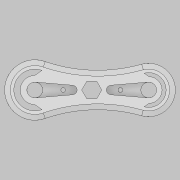
# Autodesk Inventor part: Femur_V2
Saved by Autodesk Inventor 2022.2 (Build 262287010, 287A)
## iProperties
Created: 2022-06-03
Part Number: Femur_V2
Material: Genérico
Document SubType Name: Modeling
Designer: Usuario
Density: 1 g/cm^3
Appearance: Valor por defecto
Author: Usuario
Autodesk Inventor part; units mm, degrees
ref_plane "YZ Plane" through (0, 0, 0) normal (1, 0, 0) x (0, 1, 0)
ref_plane "XZ Plane" through (0, 0, 0) normal (0, 1, 0) x (-1, 0, 0)
ref_plane "XY Plane" through (0, 0, 0) normal (0, 0, 1) x (1, 0, 0)
sketch "Boceto1" plane through (0, 0, 0) normal (0, 1, 0) x (-1, 0, 0)
  arc A0 (20.01, -12.2) -> (20.01, 12.2) centre (24.5, 0) ccw
  arc A1 (-21.2615, 11.0346) -> (-21.2615, -11.0346) centre (-24.5, 0) ccw
  line L0 (-2.1651, 3.75) -> (2.1651, 3.75)
  line L1 (2.1651, 3.75) -> (4.3301, 0)
  line L2 (4.3301, 0) -> (2.1651, -3.75)
  line L3 (2.1651, -3.75) -> (-2.1651, -3.75)
  line L4 (-2.1651, -3.75) -> (-4.3301, 0)
  line L5 (-4.3301, 0) -> (-2.1651, 3.75)
  line L6 (0, 0) -> (0, 8.5) construction
  line L7 (0, 0) -> (0, -8.5) construction
  line L8 (0, 0) -> (2.6275, 0) construction
  arc A2 (20.01, -12.2) -> (-21.4933, -11.1) centre (-2.4996, -77.9761) ccw
  arc A3 (-21.4933, 11.1) -> (20.01, 12.2) centre (-2.4996, 77.9761) ccw
  arc A4 (20.01, 12.2) -> (20.01, -12.2) centre (24.5, 0) ccw construction
  arc A5 (-21.2615, -11.0346) -> (-21.2615, 11.0346) centre (-24.5, 0) ccw construction
  point P0 (-21.4933, 11.1)
  dimension "d2" = 7.5
  dimension "d3" = 49
  dimension "d4" = 8.5
  dimension "d5" = 8.5
  dimension "d6" = 26
  dimension "d7" = 23
  dimension "d12" = 12.2
  dimension "d13" = 11.1
  constraints: 18 end point, 16 point on circle, 6 centre point, 4 symmetric about line, 2 horizontal, 2 vertical, 1 coincident, 14 other
  measures "d2" distance between parallel lines of L0 L3
  measures "d3" distance of A1.centre A0.centre
  measures "d4" distance of L6.start L6.end
  measures "d5" distance of L6.start L7.end
  measures "d6" diameter of A0
  measures "d7" diameter of A1
  measures "d12" vertical distance of A0.centre A0.start
  measures "d13" vertical distance of A1.centre A2.end
extrude "Extrusión1" add sketch "Boceto1" along normal blind 9
sketch "Boceto2" plane through (0, 9, 0) normal (0, 1, 0) x (1, 0, 0)
  arc A0 (-20.01, 12.2) -> (-20.01, -12.2) centre (-24.5, 0) ccw projected
  arc A1 (21.4933, -11.1) -> (21.4933, 11.1) centre (24.5, 0) ccw projected
  arc A2 (-24.5, 6.25) -> (-24.5, -6.25) centre (-24.5, 0) ccw
  arc A3 (24.5, -5.75) -> (24.5, 5.75) centre (24.5, 0) ccw
  arc A4 (-21.3915, 8.4462) -> (-21.3915, -8.4462) centre (-24.5, 0) ccw
  arc A5 (22.5391, -7.2391) -> (22.5391, 7.2391) centre (24.5, 0) ccw
  line L0 (-21.3915, 8.4462) -> (-24.5, 6.25)
  line L1 (-21.3915, -8.4462) -> (-24.5, -6.25)
  arc A6 (-24.5, -6.25) -> (-24.5, 6.25) centre (-24.5, 0) ccw construction
  line L2 (22.5391, 7.2391) -> (24.5, 5.75)
  line L3 (22.5391, -7.2391) -> (24.5, -5.75)
  arc A7 (24.5, 5.75) -> (24.5, -5.75) centre (24.5, 0) ccw construction
  point P0 (0, 0)
  dimension "d16" = 12.5
  dimension "d17" = 11.5
  dimension "d18" = 4
  dimension "d19" = 4
  constraints: 12 point on circle, 8 end point, 6 centre point, 2 coincident
  measures "d16" diameter of A2
  measures "d17" diameter of A3
  measures "d18" radial gap between concentric circles of A0 A4
  measures "d19" radial gap between concentric circles of A1 A5
extrude "Extrusión2" cut sketch "Boceto2" against normal up to surface (9 mm away)
sketch "Boceto3" plane through (0, 9, 0) normal (0, 1, 0) x (1, 0, 0)
  arc A0 (-24.5, 6.25) -> (-24.5, -6.25) centre (-24.5, 0) ccw projected
  arc A1 (24.5, -5.75) -> (24.5, 5.75) centre (24.5, 0) ccw projected
  arc A2 (-24.2158, 3.3881) -> (-24.2158, -3.3881) centre (-24.5, 0) ccw
  arc A3 (-8.1786, -2.0428) -> (-8.1786, 2.0428) centre (-8.35, 0) ccw
  line L0 (-27.9, 3.184) -> (-27.9, -2.3152) construction
  line L1 (-6.3, 2.5123) -> (-6.3, -1.5596) construction
  line L2 (0, 0) -> (0, -2.3152) construction
  line L3 (-24.2158, 3.3881) -> (-8.1786, 2.0428)
  line L4 (-24.2158, -3.3881) -> (-8.1786, -2.0428)
  arc A4 (24.2158, -3.3881) -> (24.2158, 3.3881) centre (24.5, 0) ccw
  arc A5 (8.1786, 2.0428) -> (8.1786, -2.0428) centre (8.35, 0) ccw
  line L5 (24.2158, 3.3881) -> (8.1786, 2.0428)
  line L6 (24.2158, -3.3881) -> (8.1786, -2.0428)
  arc A6 (-24.2158, -3.3881) -> (-24.2158, 3.3881) centre (-24.5, 0) ccw construction
  arc A7 (-8.1786, 2.0428) -> (-8.1786, -2.0428) centre (-8.35, 0) ccw construction
  arc A8 (8.1786, -2.0428) -> (8.1786, 2.0428) centre (8.35, 0) ccw construction
  arc A9 (24.2158, 3.3881) -> (24.2158, -3.3881) centre (24.5, 0) ccw construction
  dimension "d22" = 6.8
  dimension "d28" = 4.1
  dimension "d30" = 21.6
  constraints: 16 point on circle, 14 end point, 8 centre point, 6 symmetric about line, 6 tangent, 3 vertical, 1 coincident, 2 other
  measures "d22" diameter of A2
  measures "d28" diameter of A3
  measures "d30" distance between parallel lines of L0 L1
extrude "Extrusión3" cut sketch "Boceto3" against normal blind 2.5
sketch "Boceto4" plane through (0, 6.5, 0) normal (0, 1, 0) x (1, 0, 0)
  arc A0 (-24.2158, 3.3881) -> (-24.2158, -3.3881) centre (-24.5, 0) ccw projected
  line L0 (0, 0) -> (0, -3.3881) construction
  arc A1 (-24.2158, 3.3881) -> (-24.2158, -3.3881) centre (-24.5, 0) ccw projected
  circle A2 centre (-24.5, 0) radius 3.4
  circle A3 centre (-12.3, 0) radius 1
  circle A4 centre (24.5, 0) radius 3.4
  circle A5 centre (12.3, 0) radius 1
  point P0 (-24.2158, -3.3881)
  dimension "d33" = 6.8
  dimension "d34" = 2
  dimension "d35" = 12.2
  constraints: 4 centre point, 2 end point, 2 symmetric about line, 1 coincident, 1 vertical, 2 other
  measures "d33" diameter of A2
  measures "d34" diameter of A3
  measures "d35" distance of A3.centre A0.centre
extrude "Extrusión4" cut sketch "Boceto4" against normal up to surface (6.5 mm away)
sketch "Boceto5" plane through (0, 0, 0) normal (0, -1, 0) x (1, 0, 0)
  circle A0 centre (24.5, 0) radius 3.4 projected
  circle A1 centre (-24.5, 0) radius 3.4 projected
  circle A2 centre (24.5, 0) radius 9.9
  circle A3 centre (-24.5, 0) radius 10.5
  point P0 (0, 0)
  dimension "d38" = 19.8
  dimension "d39" = 21
  constraints: 2 centre point, 2 coincident
  measures "d38" diameter of A2
  measures "d39" diameter of A3
extrude "Extrusión5" cut sketch "Boceto5" against normal blind 4.1 contours A0 | A1 | A2 | A3
sketch "Boceto6" plane through (0, 0, 0) normal (0, 0, 1) x (1, 0, 0)
  line L0 (-20.01, 9) -> (21.4933, 9) projected
  line L1 (2.1651, 9) -> (-2.1651, 9) projected
  line L2 (0, 9) -> (0, 11.4954) construction
  line L3 (-37.5, 0) -> (-37.5, 9) projected
  line L4 (36, 0) -> (36, 9) projected
  line L5 (36, 0) -> (21.4933, 0) projected
  line L6 (-20.01, 0) -> (-37.5, 0) projected
  arc A0 (27, 0) -> (-28.5, 0) centre (-0.75, -126.8438) ccw
  line L7 (-9.6072, 3) -> (8.7031, 3) construction
  line L8 (-28.5, 0) -> (27, 0)
  line L9 (-20.01, 0) -> (21.4933, 0) projected
  point P0 (0, 0)
  dimension "d42" = 9
  dimension "d43" = 9
  dimension "d44" = 6
  constraints: 6 end point, 2 point on circle, 2 point on line, 1 centre point, 1 collinear, 1 horizontal, 1 midpoint, 1 tangent, 1 vertical
  measures "d42" distance from line of L3 L8.start
  measures "d43" distance from line of L4 L8.end
  measures "d44" distance between parallel lines of L0 L7
extrude "Extrusión6" cut sketch "Boceto6" along normal through all both and the other way through all
chamfer "Chaflán1" distance 2.5 angle 45 4 edges at (0.6576, 9, -8.4795) (-37.5, 9, 0) (0.6576, 9, 8.4795) (36, 9, 0)
